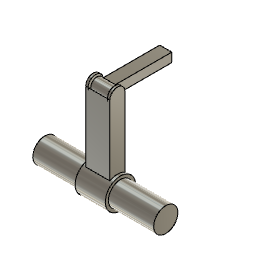
Arm1 v2 (Autodesk Fusion 360 design; units mm, degrees)
Autodesk Fusion 360 part; units mm, degrees
sketch "Sketch1" plane through (0, 0, 0) normal (1, 0, 0) x (0, 1, 0)
  circle A0 centre (0, 0) radius 40
  dimension "d5" = 80
  constraint coincident A0.centre origin
  measures "d5" diameter of A0
extrude "Extrude1" add sketch "Sketch1" along normal blind 200 and the other way blind 200 makes body 1 in component "Base Rod"
sketch "Sketch2" plane through (0, 0, 0) normal (1, 0, 0) x (0, 1, 0)
  circle A0 centre (0, 0) radius 50
  circle A1 centre (0, 0) radius 40
  dimension "d6" = 100
  constraint coincident A0.centre A1.centre
  constraint concentric A0 A1
  measures "d6" diameter of A0
extrude "Extrude1'" add sketch "Sketch2" along normal blind 50 and the other way blind 50 separate body makes body 2 in component "Arm 1"
sketch "Sketch3" plane through (0, 0, 0) normal (1, 0, 0) x (0, 1, 0)
  line L0 (0, 50) -> (0, 275)
  circle A0 centre (0, 275) radius 25
  line L1 (0, 275) -> (-60, 275)
  line L2 (-60, 275) -> (60, 275)
  line L3 (-25, 275) -> (-25, 43.3013)
  line L4 (25, 275) -> (25, 43.3013)
  circle A1 centre (0, 0) radius 50
  dimension "d19" = 225
  dimension "d20" = 50
  constraint vertical L0
  constraint coincident L0.end A0.centre
  constraint perpendicular L0 L1
  constraint perpendicular L0 L2
  constraint coincident A0 L3.start
  constraint coincident L1 L3.start
  constraint tangent A0 L3
  constraint coincident A0 L4.start
  constraint coincident L2 L4.start
  constraint tangent A0 L4
  constraint coincident A1.centre origin
  constraint coincident L0.start A1
  constraint coincident A1 L3.end
  constraint coincident A1 L4.end
  measures "d19" distance of L0.start L0.end
  measures "d20" diameter of A0
extrude "Extrude2" add sketch "Sketch3" along normal blind 40 and the other way blind 40 contours L0 A0 L3 A1 | L0 A0 L4 A1 | L0 A0 L1 L2 | L0 A0 L2 | A0 L1 L2 bodies 2 in component "Arm 1"
sketch "Sketch4" plane through (0, 0, 0) normal (1, 0, 0) x (0, 1, 0)
  line L0 (0, 50) -> (0, 275) construction
  circle A0 centre (0, 275) radius 25
  dimension "d25" = 225
  dimension "d26" = 50
  constraint vertical L0
  constraint coincident L0.end A0.centre
  measures "d25" distance of L0.start L0.end
  measures "d26" diameter of A0
extrude "Extrude3" cut sketch "Sketch4" along normal blind 32 and the other way blind 32 bodies 2 in component "Arm 1"
sketch "Sketch5" plane through (0, 0, 0) normal (1, 0, 0) x (0, 1, 0)
  line L0 (0, 50) -> (0, 275) construction
  circle A0 centre (0, 275) radius 20
  dimension "d31" = 225
  dimension "d32" = 40
  constraint vertical L0
  constraint coincident L0.end A0.centre
  measures "d31" distance of L0.start L0.end
  measures "d32" diameter of A0
extrude "Extrude1''" add sketch "Sketch5" along normal blind 28 and the other way blind 28 separate body makes body 3 in component "Arm 2"
sketch "Sketch6" plane through (0, 0, 0) normal (1, 0, 0) x (0, 1, 0)
  line L0 (0, 295) -> (0, 290) construction
  line L1 (13.0091, 290) -> (200, 290)
  line L2 (0, 255) -> (0, 260) construction
  line L3 (13.0091, 260) -> (200, 260)
  line L4 (200, 260) -> (200, 290)
  circle A0 centre (0, 275) radius 19.8554
  dimension "d41" = 5
  dimension "d42" = 200
  dimension "d43" = 5
  dimension "d44" = 200
  constraint vertical L0
  constraint perpendicular L0 L1
  constraint perpendicular L1 L2
  constraint perpendicular L2 L3
  constraint perpendicular L1 L4
  constraint coincident A0 L1.start
  constraint coincident A0 L3.start
  measures "d41" distance of L0.start L0.end
  measures "d42" distance of L0.end L1.end
  measures "d43" distance of L2.start L2.end
  measures "d44" distance of L2.end L3.end
extrude "Extrude2'" add sketch "Sketch6" along normal blind 20 and the other way blind 20 contours L1 L3 L4 A0 bodies 3 in component "Arm 2"
sketch "Sketch7" plane through (0, 25, 0) normal (0, 1, 0) x (-1, 0, 0)
  line L0 (40, 275) -> (32, 275)
  line L1 (32, 275) -> (-32, 275)
  line L2 (-32, 275) -> (-40, 275)
  line L3 (-40, 275) -> (-40, 43.3013)
  line L4 (-40, 43.3013) -> (40, 43.3013)
  line L5 (40, 43.3013) -> (40, 275)
  line L6 (-19.9929, 275) -> (-19.9929, 75)
  line L7 (20, 275) -> (20, 75)
  line L8 (20, 75) -> (-19.9929, 75)
  dimension "d49" = 200
  dimension "d50" = 200
  constraint coincident L1 L6.start
  constraint perpendicular L1 L6
  constraint coincident L1 L7.start
  constraint perpendicular L1 L7
  measures "d49" distance of L6.start L6.end
  measures "d50" distance of L7.start L7.end
extrude "Extrude3'" [suppressed] in component "Arm 2"
extrude "Extrude4" cut sketch "Sketch7" along normal blind -15 and the other way blind -20 contours L1 L6 L7 L8 bodies 2 in component "Arm 1"
sketch "Sketch8" plane through (-32, 0, 0) normal (1, 0, 0) x (0, 1, 0)
  arc A0 (25, 275) -> (-25, 275) centre (0, 275) ccw
  arc A1 (-25, 275) -> (25, 275) centre (0, 275) ccw
  circle A2 centre (0, 275) radius 5
  constraint concentric A0 A2
extrude "Extrude5" cut sketch "Sketch8" along normal blind 66 and the other way blind 2 contours A2 bodies 2 in component "Arm 1"
extrude "Extrude4'" cut sketch "Sketch8" along normal blind 66 and the other way blind 2 contours A2 sketch seen with x (1, 0, 0) y (0, 0.906308, 0.422618) z (0, -0.422618, 0.906308) at (0, 116.22, 25.7654) bodies 3 in component "Arm 2"
sketch "Sketch9" plane through (-34, 0, 0) normal (1, 0, 0) x (0, 1, 0)
  circle A0 centre (0, 275) radius 5
  circle A1 centre (0, 275) radius 3
  constraint concentric A0 A1
extrude "Extrude1'''" add sketch "Sketch9" along normal up to surface (68 mm away) separate body contours A1 makes body 4 in component "Component"
component "Base Rod" placed x (1, 0, 0) y (0, 1, 0) z (0, 0, 1) at (0, 0, 0)
component "Arm 1" placed x (1, 0, 0) y (0, 1, 0) z (0, 0, 1) at (0, 0, 0)
component "Arm 2" placed x (1, 0, 0) y (0, 1, 0) z (0, 0, 1) at (0, 0, 0)
component "Component" placed x (1, 0, 0) y (0, 1, 0) z (0, 0, 1) at (0, 0, 0)
named bodies: "Arm 1", "Arm 2"
